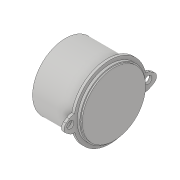
# Autodesk Inventor part: PIEZO
Saved by Autodesk Inventor 2019 (Build 230136000, 136)
## iProperties
Created: 2019-11-28
Part Number: PIEZO
Material: Generic
Document SubType Name: Modeling
Designer: Abhishek
Density: 1 g/cm^3
Appearance: Default
Author: Abhishek
Autodesk Inventor part; units mm, degrees
ref_plane "YZ Plane" through (0, 0, 0) normal (1, 0, 0) x (0, 1, 0)
ref_plane "XZ Plane" through (0, 0, 0) normal (0, 1, 0) x (-1, 0, 0)
ref_plane "XY Plane" through (0, 0, 0) normal (0, 0, 1) x (1, 0, 0)
sketch "Sketch1" plane through (0, 0, 0) normal (1, 0, 0) x (0, 1, 0)
  circle A0 centre (0, 0) radius 12.5
  dimension "d0" = 25
  constraints: 1 centre point, 1 coincident
  measures "d0" diameter of A0
extrude "Extrusion1" add sketch "Sketch1" along normal blind 16
sketch "Sketch2" plane through (16, 0, 0) normal (1, 0, 0) x (0, 0, -1)
  circle A0 centre (0, 0) radius 13.8287
  arc A1 (-13.5463, 2.7804) -> (-13.3988, -3.4214) centre (-13.6396, -0.3245) ccw
  arc A2 (13.3988, -3.4214) -> (13.5463, 2.7804) centre (13.6137, -0.3239) ccw
  line L0 (-15.4609, 2.1919) -> (-18.4894, 0)
  arc A3 (-18.4894, 0) -> (-15.4609, -2.8409) centre (-9.6242, 6.4162) ccw
  line L1 (15.4336, 2.1919) -> (18.879, 0)
  arc A4 (15.4336, -2.8396) -> (18.879, 0) centre (12.797, 3.8693) ccw
  constraints: 16 point on circle, 5 centre point, 4 end point, 2 point on line, 1 coincident, 1 tangent
extrude "Extrusion2" add sketch "Sketch2" along normal blind 1
fillet "Fillet1" radius 2 2 edges at (16.5, 0, 18.4894) (16.5, 0, -18.879)
sketch "Sketch3" plane through (17, 0, 0) normal (1, 0, 0) x (0, 0, -1)
  circle A0 centre (0, 0) radius 12.5
  constraints: 1 centre point, 1 coincident
extrude "Extrusion3" add sketch "Sketch3" along normal blind 1
sketch "Sketch4" plane through (17, 0, 0) normal (1, 0, 0) x (0, 0, -1)
  circle A0 centre (-15.0948, 0) radius 1.3586
  circle A1 centre (14.6009, 0) radius 1.4082
  point P0 (0, 0)
  constraints: 2 centre point
extrude "Extrusion4" cut sketch "Sketch4" against normal blind 1
sketch "Sketch5" plane through (18, 0, 0) normal (1, 0, 0) x (0, 0, -1)
  point P0 (0, 0)
sketch "Sketch6" plane through (18, 0, 0) normal (1, 0, 0) x (0, 0, -1)
  circle A0 centre (0, 0) radius 12.0611
  constraints: 1 centre point, 1 coincident
extrude "Extrusion5" add sketch "Sketch6" along normal blind 0.5
body "Solid1"
